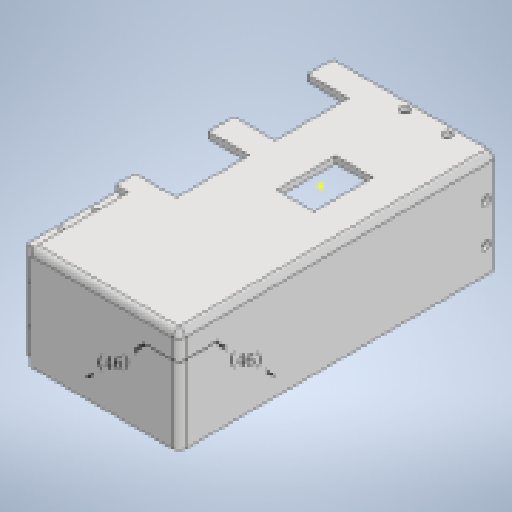
# Autodesk Inventor part: top_3
Saved by Autodesk Inventor 2023 (Build 270158000, 158)
## iProperties
Created: 2024-04-26
Part Number: top_3
Material: 常规
Document SubType Name: Modeling
Designer: Nitrene.P.L
Density: 1 g/cm^3
Appearance: 默认
Author: Nitrene.P.L
Autodesk Inventor part; units mm, degrees
ref_plane "YZ Plane" through (0, 0, 0) normal (1, 0, 0) x (0, 1, 0)
ref_plane "XZ Plane" through (0, 0, 0) normal (0, 1, 0) x (-1, 0, 0)
ref_plane "XY Plane" through (0, 0, 0) normal (0, 0, 1) x (1, 0, 0)
sketch "草图5" plane through (0, 0, 0) normal (0, 1, 0) x (-1, 0, 0)
  line L0 (125, 235) -> (-125, 235)
  line L1 (-125, 235) -> (-125, -235)
  line L2 (-125, -235) -> (125, -235)
  line L3 (125, -235) -> (125, 235)
  line L4 (0, 3) -> (0, -5)
  line L5 (3.5058, 0) -> (-3.4421, 0)
  line L6 (25, 144) -> (-32, 144)
  line L7 (-32, 144) -> (-32, 87)
  line L8 (-32, 87) -> (25, 87)
  line L9 (25, 87) -> (25, 144)
  line L10 (25, 67) -> (-32, 67)
  line L11 (-32, 67) -> (-32, 10)
  line L12 (-32, 10) -> (25, 10)
  line L13 (25, 10) -> (25, 67)
  line L14 (25, -10) -> (-32, -10)
  line L15 (-32, -10) -> (-32, -67)
  line L16 (-32, -67) -> (25, -67)
  line L17 (25, -67) -> (25, -10)
  line L18 (25, -87) -> (-32, -87)
  line L19 (-32, -87) -> (-32, -144)
  line L20 (-32, -144) -> (25, -144)
  line L21 (25, -144) -> (25, -87)
  line L22 (-66, 100) -> (-95, 100)
  line L23 (-95, 100) -> (-95, 54)
  line L24 (-95, 54) -> (-66, 54)
  line L25 (-66, 54) -> (-66, 100)
  line L26 (-66, -54) -> (-95, -54)
  line L27 (-95, -54) -> (-95, -100)
  line L28 (-95, -100) -> (-66, -100)
  line L29 (-66, -100) -> (-66, -54)
  line L30 (100, 15) -> (70, 15)
  line L31 (70, 15) -> (70, -15)
  line L32 (70, -15) -> (100, -15)
  line L33 (100, -15) -> (100, 15)
  circle A0 centre (65, 182) radius 10
  circle A1 centre (65, -182) radius 10
  circle A2 centre (65, 182) radius 15
  circle A3 centre (80, 182) radius 1.5
  circle A4 centre (57.5, 194.9904) radius 1.5
  circle A5 centre (57.5, 169.0096) radius 1.5
  line L34 (125, 235) -> (0, 235)
  line L35 (0, 235) -> (0, 0)
  line L36 (0, 0) -> (125, 0)
  line L37 (125, 0) -> (125, 235)
  line L38 (-125, 235) -> (0, 235)
  line L39 (0, 235) -> (0, 0)
  line L40 (0, 0) -> (-125, 0)
  line L41 (-125, 0) -> (-125, 235)
  line L42 (-125, -235) -> (0, -235)
  line L43 (0, -235) -> (0, 0)
  line L44 (0, 0) -> (-125, 0)
  line L45 (-125, 0) -> (-125, -235)
  line L46 (125, -235) -> (0, -235)
  line L47 (0, -235) -> (0, 0)
  line L48 (0, 0) -> (125, 0)
  line L49 (125, 0) -> (125, -235)
  circle A6 centre (65, -182) radius 15
  circle A7 centre (80, -182) radius 1.5
  circle A8 centre (57.5, -169.0096) radius 1.5
  circle A9 centre (57.5, -194.9904) radius 1.5
  point P0 (0, 67)
  point P1 (0, 87)
  point P2 (0, 144)
  point P3 (0, 10)
  dimension "d142" = 30
  dimension "d145" = 30
  dimension "d111" = 470
  dimension "d112" = 250
  dimension "d113" = 57
  dimension "d114" = 57
  dimension "d115" = 57
  dimension "d116" = 57
  dimension "d117" = 57
  dimension "d118" = 57
  dimension "d119" = 57
  dimension "d120" = 57
  dimension "d121" = 91
  dimension "d122" = 20
  dimension "d123" = 20
  dimension "d124" = 20
  dimension "d125" = 93
  dimension "d126" = 29
  dimension "d127" = 46
  dimension "d128" = 46
  dimension "d129" = 135
  dimension "d130" = 108
  dimension "d131" = 30
  dimension "d132" = 30
  dimension "d133" = 30
  dimension "d134" = 25
  dimension "d135" = 220
  dimension "d136" = 20
  dimension "d137" = 53
  dimension "d138" = 60
  dimension "d139" = 20
  dimension "d140" = 53
  dimension "d141" = 60
  dimension "d143" = 3
  dimension "d144" = 360
  dimension "d146" = 3
  dimension "d147" = 360
  constraints: 100 end point, 24 parallel, 14 horizontal, 12 perpendicular, 8 centre point, 3 collinear, 2 coincident, 2 horizontal alignment, 2 point on line, 2 vertical, 20 other
  measures "d111" distance of L3.start L0.start
  measures "d112" distance of L0.start L0.end
  measures "d113" distance of L9.start L8.start
  measures "d114" distance of L8.start L6.end
  measures "d115" distance of L13.start L12.start
  measures "d116" distance of L12.start L10.end
  measures "d117" distance of L17.start L16.start
  measures "d118" distance of L16.start L15.start
  measures "d119" distance of L21.start L20.start
  measures "d120" distance of L20.start L18.end
  measures "d121" distance between parallel lines of L0 L6
  measures "d122" distance between parallel lines of L10 L8
  measures "d123" distance between parallel lines of L12 L14
  measures "d124" distance between parallel lines of L18 L16
  measures "d125" distance between parallel lines of L1 L7
  measures "d126" distance of L25.start L24.start
  measures "d127" distance of L24.start L23.start
  measures "d128" distance of L28.start L26.end
  measures "d129" distance between parallel lines of L0 L22
  measures "d130" distance between parallel lines of L26 L24
  measures "d131" distance between parallel lines of L1 L23
  measures "d132" distance of L32.end L32.start
  measures "d133" distance of L32.start L31.start
  measures "d134" distance between parallel lines of L3 L33
  measures "d135" distance between parallel lines of L0 L30
  measures "d136" diameter of A0
  measures "d137" distance from line of L0 A0.centre
  measures "d138" distance from line of L3 A0.centre
  measures "d139" diameter of A1
  measures "d140" distance from line of L2 A1.centre
  measures "d141" distance from line of L3 A1.centre
  measures "d143" diameter of A3
  measures "d146" diameter of A7
extrude "拉伸5" add sketch "草图5" along normal blind 10 contours L35 L6 L7 L8 L10 L11 L12 L4 L5 L40 L1 L0
sketch "草图6" plane through (0, 0, 0) normal (0, -1, 0) x (1, 0, 0)
  line L0 (125, 0) -> (0, 0) projected
  line L1 (0, 144) -> (0, 235) projected
  line L2 (47, 0) -> (0, 0)
  line L3 (0, 0) -> (0, 159)
  line L4 (0, 159) -> (47, 159)
  line L5 (47, 159) -> (47, 0)
  line L6 (32, 87) -> (32, 144) projected
  line L7 (32, 144) -> (0, 144) projected
  line L8 (111, 115) -> (47, 115)
  line L9 (47, 115) -> (47, 39)
  line L10 (47, 39) -> (111, 39)
  line L11 (111, 39) -> (111, 115)
  line L12 (95, 54) -> (95, 100) projected
  line L13 (95, 100) -> (66, 100) projected
  line L14 (66, 54) -> (95, 54) projected
  line L15 (66, 100) -> (66, 54) projected
  dimension "d150" = 15
  dimension "d151" = 15
  dimension "d152" = 16
  dimension "d153" = 15
  dimension "d154" = 15
  dimension "d155" = 19
  constraints: 16 end point, 4 parallel, 2 horizontal, 2 perpendicular, 2 point on line
  measures "d150" distance between parallel lines of L6 L5
  measures "d151" distance between parallel lines of L7 L4
  measures "d152" distance between parallel lines of L12 L11
  measures "d153" distance between parallel lines of L8 L13
  measures "d154" distance between parallel lines of L10 L14
  measures "d155" distance between parallel lines of L15 L9
extrude "拉伸6" cut sketch "草图6" against normal blind 5 contours L0 L3 L1 L4 L5 | L5 L8 L11 L10 | L14 L15 L13 L12
sketch "草图7" plane through (0, 10, 0) normal (0, 1, 0) x (1, 0, 0)
  line L0 (0, -144) -> (0, -159) projected
  line L1 (0, -235) -> (125, -235) projected
  line L2 (0, -159) -> (10, -159)
  line L3 (10, -159) -> (10, -235)
  line L4 (10, -235) -> (0, -235)
  line L5 (0, -235) -> (0, -159)
  point P0 (0, 0)
  dimension "d158" = 10
  constraints: 8 end point, 2 parallel, 1 horizontal, 1 perpendicular, 1 point on line
  measures "d158" distance of L3.end L4.end
extrude "拉伸7" cut sketch "草图7" against normal blind 5
sketch "草图8" plane through (0, 5, 0) normal (0, 1, 0) x (1, 0, 0)
  circle A0 centre (4, -205) radius 2.1
  circle A1 centre (4, -179) radius 2.1
  line L0 (0, -235) -> (0, -159) projected
  line L1 (10, -235) -> (0, -235) projected
  line L2 (32, -144) -> (0, -144) projected
  line L3 (0, -159) -> (10, -159) projected
  point P0 (0, 0)
  dimension "d161" = 4.2
  dimension "d162" = 4.2
  dimension "d163" = 4
  dimension "d164" = 4
  dimension "d165" = 30
  dimension "d169" = 20
  constraints: 2 centre point
  measures "d161" diameter of A0
  measures "d162" diameter of A1
  measures "d163" distance from line of L0 A0.centre
  measures "d164" distance from line of A1.centre L0
  measures "d165" distance from line of L1 A0.centre
  measures "d169" distance from line of L3 A1.centre
extrude "拉伸8" cut sketch "草图8" against normal blind 5
sketch "草图9" plane through (0, 0, 0) normal (0, -1, 0) x (1, 0, 0)
  line L0 (125, 0) -> (0, 0) projected
  line L1 (0, 235) -> (125, 235) projected
  line L2 (125, 0) -> (111, 0)
  line L3 (111, 0) -> (111, 235)
  line L4 (111, 235) -> (125, 235)
  line L5 (125, 235) -> (125, 0)
  line L6 (0, 159) -> (0, 235) projected
  line L7 (125, 235) -> (125, 0) projected
  line L8 (0, 235) -> (125, 235)
  line L9 (125, 235) -> (125, 221)
  line L10 (125, 221) -> (0, 221)
  line L11 (0, 221) -> (0, 235)
  point P0 (0, 221)
  point P1 (111, 221)
  dimension "d170" = 14
  dimension "d171" = 14
  constraints: 16 end point, 4 parallel, 2 horizontal, 2 perpendicular, 2 point on line
  measures "d170" distance of L3.end L4.end
  measures "d171" distance of L8.end L9.end
extrude "拉伸9" add sketch "草图9" along normal blind 70
sketch "草图10" plane through (10, 10, 235) normal (0, 0, 1) x (1, 0, 0)
  line L0 (0, -5) -> (-10, -5) projected
  line L1 (-10, -80) -> (-10, -5) projected
  line L2 (0, -5) -> (-10, -5)
  line L3 (-10, -5) -> (-10, -80)
  line L4 (-10, -80) -> (0, -80)
  line L5 (0, -80) -> (0, -5)
  point P0 (-10, -10)
  constraints: 8 end point, 2 parallel, 1 horizontal, 1 perpendicular
extrude "拉伸10" cut sketch "草图10" against normal blind 7
sketch "草图11" plane through (10, 10, 228) normal (0, 0, 1) x (1, 0, 0)
  circle A0 centre (-6, -30) radius 2.1
  circle A1 centre (-6, -60) radius 2.1
  line L0 (-10, -80) -> (-10, -5) projected
  line L1 (0, -80) -> (-10, -80) projected
  line L2 (0, 0) -> (115, 0) projected
  point P0 (-10, -10)
  dimension "d176" = 4.2
  dimension "d177" = 4.2
  dimension "d178" = 4
  dimension "d179" = 4
  dimension "d180" = 20
  dimension "d181" = 30
  constraints: 2 centre point
  measures "d176" diameter of A0
  measures "d177" diameter of A1
  measures "d178" distance from line of L0 A0.centre
  measures "d179" distance from line of L0 A1.centre
  measures "d180" distance from line of L1 A1.centre
  measures "d181" distance from line of L2 A0.centre
extrude "拉伸11" cut sketch "草图11" against normal blind 7
fillet "圆角2" radius 10 4 edges at (111, 0, 168) (111, 0, 19.5) (111, -35, 221) (55.5, 0, 221)
sketch "草图12" plane through (0, 0, 0) normal (0, -1, 0) x (1, 0, 0)
  circle A0 centre (65, 175) radius 10
  line L0 (125, 0) -> (125, 235) projected
  line L1 (125, 235) -> (10, 235) projected
  point P0 (0, 0)
  point P1 (125, 230)
  point P2 (120, 235)
  dimension "d186" = 20
  dimension "d187" = 60
  dimension "d188" = 60
  constraints: 1 centre point
  measures "d186" diameter of A0
  measures "d187" distance from line of L0 A0.centre
  measures "d188" distance from line of L1 A0.centre
extrude "拉伸12" add sketch "草图12" along normal blind 70
fillet "圆角3" radius 10 1 edges at (55, 0, 175)
sketch "草图14" plane through (125, 10, 235) normal (1, 0, 0) x (0, 0, -1)
  line L0 (235, -80) -> (235, 0) projected
  line L1 (235, 0) -> (245, 0)
  line L2 (245, 0) -> (245, -80)
  line L3 (245, -80) -> (235, -80)
  line L4 (235, -80) -> (235, 0)
  line L5 (0, 0) -> (235, 0) projected
  circle A0 centre (239, -60) radius 2.1
  circle A1 centre (239, -30) radius 2.1
  point P0 (235, -10)
  dimension "d192" = 10
  dimension "d193" = 80
  dimension "d196" = 4.2
  dimension "d197" = 4.2
  dimension "d198" = 6
  dimension "d199" = 6
  dimension "d200" = 20
  dimension "d201" = 30
  constraints: 8 end point, 2 centre point, 2 parallel, 1 horizontal, 1 perpendicular
  measures "d192" distance of L2.end L3.end
  measures "d193" distance between parallel lines of L5 L3
  measures "d196" diameter of A0
  measures "d197" diameter of A1
  measures "d198" distance from line of L2 A0.centre
  measures "d199" distance from line of L2 A1.centre
  measures "d200" distance from line of L3 A0.centre
  measures "d201" distance from line of L1 A1.centre
extrude "拉伸14" add sketch "草图14" against normal blind 7
sketch "草图15" plane through (0, 10, 0) normal (0, 1, 0) x (1, 0, 0)
  line L0 (118, 0) -> (0, 0)
  circle A0 centre (95, 4) radius 2.1
  circle A1 centre (62, 4) radius 2.1
  line L1 (125, -235) -> (125, 10) projected
  line L2 (118, 0) -> (32, 0)
  line L3 (32, 0) -> (32, 10)
  line L4 (32, 10) -> (118, 10)
  line L5 (118, 10) -> (118, 0)
  line L6 (32, -10) -> (32, -67) projected
  line L7 (125, 10) -> (118, 10) projected
  point P0 (32, 0)
  dimension "d205" = 4.2
  dimension "d206" = 4.2
  dimension "d209" = 30
  dimension "d212" = 6
  dimension "d213" = 6
  dimension "d214" = 30
  constraints: 10 end point, 2 centre point, 2 collinear, 2 horizontal, 2 parallel, 1 perpendicular
  measures "d205" diameter of A0
  measures "d206" diameter of A1
  measures "d209" distance from line of L1 A0.centre
  measures "d212" distance from line of L4 A0.centre
  measures "d213" distance from line of L4 A1.centre
  measures "d214" distance from line of L3 A1.centre
extrude "拉伸15" add sketch "草图15" against normal blind 5
sketch "草图16" plane through (0, 10, 0) normal (0, 1, 0) x (1, 0, 0)
  circle A0 centre (95, 4) radius 2.1 projected
  circle A1 centre (95, 4) radius 3.6
  circle A2 centre (62, 4) radius 2.1 projected
  circle A3 centre (62, 4) radius 3.6
  point P0 (0, 0)
  dimension "d217" = 7.2
  dimension "d218" = 7.2
  constraints: 2 centre point, 2 coincident
  measures "d217" diameter of A1
  measures "d218" diameter of A3
extrude "拉伸16" cut sketch "草图16" against normal blind 4
sketch "草图17" plane through (125, -70, 235) normal (1, 0, 0) x (0, 0, -1)
  circle A0 centre (239, 50) radius 2.1 projected
  circle A1 centre (239, 50) radius 3.6
  circle A2 centre (239, 20) radius 2.1 projected
  circle A3 centre (239, 20) radius 3.6
  point P0 (235, 70)
  dimension "d221" = 7.2
  dimension "d222" = 7.2
  constraints: 2 centre point, 2 coincident
  measures "d221" diameter of A1
  measures "d222" diameter of A3
extrude "拉伸17" cut sketch "草图17" against normal blind 4
fillet "圆角4" radius 5 3 edges at (125, 10, 112.5) (67.5, 10, 235) (125, -30, 235)
sketch "草图18" plane through (0, 10, 0) normal (0, 1, 0) x (1, 0, 0)
  line L0 (0, 0) -> (0, -10) projected
  line L1 (32, 10) -> (118, 10) projected
  line L2 (0, 0) -> (32, 0)
  line L3 (32, 0) -> (32, 10)
  line L4 (32, 10) -> (0, 10)
  line L5 (0, 10) -> (0, 0)
  constraints: 8 end point, 2 parallel, 1 horizontal, 1 perpendicular
extrude "拉伸18" add sketch "草图18" against normal blind 5
sketch "草图20" plane through (0, -70, 0) normal (0, -1, 0) x (1, 0, 0)
  circle A0 centre (65, 175) radius 10 projected
  circle A1 centre (65, 175) radius 10
  line L0 (111, 211) -> (111, 0) projected
  line L1 (0, 221) -> (101, 221) projected
  point P0 (0, 0)
  dimension "d228" = 46
  dimension "d229" = 46
  constraints: 1 centre point, 1 coincident
  measures "d228" distance from line of L0 A1.centre
  measures "d229" distance from line of L1 A1.centre
